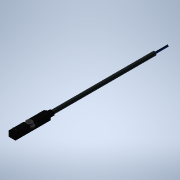
# Autodesk Inventor part: 574333 SMT-8M-A-1---OE---(part)
Saved by Autodesk Inventor 2021 (Build 250183000, 183)
## iProperties
Created: 2026-04-08
Part Number: 574333 SMT-8M-A-1---OE---(part)
Material: Generic
Catalog Web Link: www.3dfindit.com
Description: SMT-8M-A_part-Proximity switch
Vendor: FESTO
Document SubType Name: Modeling
Designer: psAdmin
Manufacturer: FESTO
Mass: 1.11911 g
Surface Area: 14.2957 cm^2
Volume: 1.11911 cm^3
Density: 1 g/cm^3
Appearance: PSOLRGB-176-176-176
Category: PARTsolutions
Company: FESTO
Title: 574333 SMT-8M-A-1---OE---(part)
Author: Cadenas PARTsolutions
Comments: Proximity switch
PSOL_IDENT_0: {$CADENAS_DATA/23d-libs/festo/parts/s/smt/parts/smt_8m_a.prj},219 {VTYP=3D},{NB=574333 SMT-8M-A-1---
PSOL_IDENT_1: OE---(part)},{LINA=574333 SMT-8M-A-1---OE---(part)},{NN=SMT-8M-A_part},{DATE=22.11.2021 21:11:07},{G
PSOL_IDENT_2: EOMDATE=22.11.2021 21:11:00},{VERSION=},{LINEID=10},{WBVAR=SA,LB,AT},{WBNUMERIC=SA}  {NB=574333 SMT-
PSOL_IDENT_3: 8M-A-1---OE---(part)},{LINA=574333 SMT-8M-A-1---OE---(part)},{KT=DUMMY},{TNR=574333},{TYP=SMT-8M-A},
PSOL_IDENT_4: {SA=1},{LB=-},{AT=OE}
NB: 574333 SMT-8M-A-1---OE---(part)
NN: SMT-8M-A_part
NT: Proximity switch
NBSYN: $TNR. $TYP.-$SA.-$LB.-$AT.---(part)
LINA: 574333 SMT-8M-A-1---OE---(part)
CATALOG: Festo
TNR: 574333
TYP: SMT-8M-A
SA: PS
LB: -
AT: OE
SUPPLIER: FESTO
ARTICLENO: 574333 SMT-8M-A-1---OE---(part)
BOMINFO: 574333 SMT-8M-A-1---OE---(part)
CREATOR: CADENAS GmbH
Autodesk Inventor part; units mm, degrees
sketch "Sketch_1" plane through (0, 0, 0) normal (0, 0, 1) x (1, 0, 0)
  line L0 (-2.5, 4.0386) -> (-2.5, 0)
  line L1 (-2.5, 0) -> (2.5, 0)
  line L2 (2.5, 0) -> (2.5, 4.0386)
  arc A0 (2.5, 4.0386) -> (2.3613, 4.229) centre (2.3, 4.0386) ccw
  arc A1 (2.3613, 4.229) -> (-2.3613, 4.229) centre (0, -3.1) ccw
  arc A2 (-2.3613, 4.229) -> (-2.5, 4.0386) centre (-2.3, 4.0386) ccw
  constraints: 6 end point, 6 point on circle, 3 centre point
extrude "Extrusion1" add sketch "Sketch_1" along normal blind 26.3
sketch "Sketch_2" plane through (-1.6, 0, 0) normal (1, 0, 0) x (0, 0, -1)
  line L0 (-15.3, 3.85) -> (-15.3, 2)
  line L1 (-15.3, 2) -> (-10.025, 2)
  line L2 (-10.025, 2) -> (-10.025, 3.15)
  line L3 (-10.025, 3.15) -> (-10.725, 3.15)
  line L4 (-10.725, 3.15) -> (-10.725, 3.85)
  line L5 (-10.725, 3.85) -> (-15.3, 3.85)
  constraints: 12 end point
extrude "Extrusion2" cut sketch "Sketch_2" along normal blind 4.1
sketch "Sketch_3" plane through (-2.5, 0, 0) normal (1, 0, 0) x (0, 0, -1)
  line L0 (-16.875, 3.85) -> (-16.875, 2)
  line L1 (-16.875, 2) -> (-11.6, 2)
  line L2 (-11.6, 2) -> (-11.6, 3.85)
  line L3 (-11.6, 3.85) -> (-16.875, 3.85)
  constraints: 8 end point
extrude "Extrusion3" cut sketch "Sketch_3" along normal blind 4.1
sketch "Sketch_4" plane through (0, 4.6, 0) normal (0, 1, 0) x (1, 0, 0)
  line L0 (-3, -15.3) -> (-1.3666, -15.3)
  arc A0 (-1.3666, -15.3) -> (1.3666, -15.3) centre (0, -13.45) ccw
  line L1 (1.3666, -15.3) -> (3, -15.3)
  line L2 (3, -15.3) -> (3, -11.6)
  line L3 (3, -11.6) -> (1.3666, -11.6)
  arc A1 (1.3666, -11.6) -> (-1.3666, -11.6) centre (0, -13.45) ccw
  line L4 (-1.3666, -11.6) -> (-3, -11.6)
  line L5 (-3, -11.6) -> (-3, -15.3)
  constraints: 12 end point, 4 point on circle, 2 centre point
extrude "Extrusion4" cut sketch "Sketch_4" against normal blind 2.5
sketch "Sketch_5" plane through (0, 2, 0) normal (0, 1, 0) x (1, 0, 0)
  arc A0 (-2.6719, -11.644) -> (-2.6719, -15.256) centre (0, -13.45) ccw
  arc A1 (-2.6719, -15.256) -> (-2.589, -15.3) centre (-2.589, -15.2) ccw
  line L0 (-2.589, -15.3) -> (-1.9442, -15.3)
  arc A2 (-1.6255, -15.4148) -> (-1.9442, -15.3) centre (-1.9442, -15.8) ccw
  arc A3 (-1.6255, -15.4148) -> (1.6255, -15.4148) centre (0, -13.45) ccw
  arc A4 (1.9442, -15.3) -> (1.6255, -15.4148) centre (1.9442, -15.8) ccw
  line L1 (1.9442, -15.3) -> (2.589, -15.3)
  arc A5 (2.589, -15.3) -> (2.6719, -15.256) centre (2.589, -15.2) ccw
  arc A6 (2.6719, -15.256) -> (2.6719, -11.644) centre (0, -13.45) ccw
  arc A7 (2.6719, -11.644) -> (2.589, -11.6) centre (2.589, -11.7) ccw
  line L2 (2.589, -11.6) -> (1.9442, -11.6)
  arc A8 (1.6255, -11.4852) -> (1.9442, -11.6) centre (1.9442, -11.1) ccw
  arc A9 (1.6255, -11.4852) -> (-1.6255, -11.4852) centre (0, -13.45) ccw
  arc A10 (-1.9442, -11.6) -> (-1.6255, -11.4852) centre (-1.9442, -11.1) ccw
  line L3 (-1.9442, -11.6) -> (-2.589, -11.6)
  arc A11 (-2.589, -11.6) -> (-2.6719, -11.644) centre (-2.589, -11.7) ccw
  constraints: 24 point on circle, 12 centre point, 8 end point
extrude "Extrusion5" add sketch "Sketch_5" along normal blind 1
sketch "Sketch_6" plane through (0, 0, 13.45) normal (0, 0, 1) x (1, 0, 0)
  line L0 (0, 2) -> (0, 4.6)
  line L1 (0, 4.6) -> (2.25, 4.6)
  line L2 (2.25, 4.6) -> (2.25, 3.9)
  line L3 (2.25, 3.9) -> (1.6935, 3.9)
  line L4 (1.6935, 3.9) -> (1.6935, 3.6)
  line L5 (1.6935, 3.6) -> (2, 3.2935)
  line L6 (2, 3.2935) -> (2, 2.3065)
  line L7 (2, 2.3065) -> (1.6935, 2)
  line L8 (1.6935, 2) -> (0, 2)
  line L9 (0, 2) -> (0, 4.6)
  constraints: 20 end point
revolve "Revolution1" add sketch "Sketch_6" angle 360 about axis through (0, 2, 13.45) along (0, -1, 0)
thread "Thread1" size "M4x0.5" class "6g" standard "ISO Metric profile" length 0.987
sketch "Sketch_7" plane through (0, 4.6, 13.45) normal (0, 1, 0) x (1, 0, 0)
  line L0 (-0.75, -0.433) -> (0, -0.866)
  line L1 (0, -0.866) -> (0.75, -0.433)
  line L2 (0.75, -0.433) -> (0.75, 0.433)
  line L3 (0.75, 0.433) -> (0, 0.866)
  line L4 (0, 0.866) -> (-0.75, 0.433)
  line L5 (-0.75, 0.433) -> (-0.75, -0.433)
  constraints: 12 end point
extrude "Extrusion6" cut sketch "Sketch_7" against normal blind 1.4
sketch "Sketch_9" plane through (0, 0, 23.21) normal (0, 0, 1) x (1, 0, 0)
  line L0 (-2.5, 2.8) -> (2.5, 2.8)
  line L1 (2.5, 2.8) -> (2.5, 4.2485)
  arc A0 (2.5, 4.2485) -> (2.3597, 4.4393) centre (2.3, 4.2485) ccw
  arc A1 (2.3597, 4.4393) -> (-2.3597, 4.4393) centre (0, -3.1) ccw
  arc A2 (-2.3597, 4.4393) -> (-2.5, 4.2485) centre (-2.3, 4.2485) ccw
  line L2 (-2.5, 4.2485) -> (-2.5, 2.8)
  constraints: 6 end point, 6 point on circle, 3 centre point
extrude "Extrusion7" add sketch "Sketch_9" along normal mid plane 0.4
sketch "Sketch_10" plane through (0, 0, 23.21) normal (0, 0, 1) x (1, 0, 0)
  line L0 (-0.2, 2.78) -> (0.2, 2.78)
  line L1 (0.2, 2.78) -> (0.2, 4.78)
  line L2 (0.2, 4.78) -> (-0.2, 4.78)
  line L3 (-0.2, 4.78) -> (-0.2, 2.78)
  constraints: 8 end point
extrude "Extrusion8" add sketch "Sketch_10" along normal mid plane 2
sketch "Sketch_11" plane through (0, 0, 0) normal (1, 0, 0) x (0, 1, 0)
  line L0 (2.05, -90) -> (2.05, 0)
  line L1 (2.05, 0) -> (4.05, 0)
  line L2 (4.05, 0) -> (4.05, -3)
  line L3 (4.05, -3) -> (3.5, -3)
  line L4 (3.5, -3) -> (3.5, -90)
  line L5 (3.5, -90) -> (2.05, -90)
  line L6 (2.05, -90) -> (2.05, 0)
  constraints: 14 end point
revolve "Revolution2" add sketch "Sketch_11" angle 360 about axis through (0, 2.05, -90) along (0, 0, -1)
sketch "Sketch_12" plane through (0, 2.05, -90) normal (0, 0, -1) x (0, 1, 0)
  line L0 (-2, -2) -> (2, -2)
  line L1 (2, -2) -> (2, 2)
  line L2 (2, 2) -> (-2, 2)
  line L3 (-2, 2) -> (-2, -2)
  circle A0 centre (0.4, 0) radius 0.3
  circle A1 centre (-0.2, 0.3464) radius 0.3
  circle A2 centre (-0.2, -0.3464) radius 0.3
  constraints: 8 end point, 3 centre point
extrude "Extrusion9" cut sketch "Sketch_12" against normal blind 10
sketch "Sketch_17" plane through (0, 0, -1.5) normal (0, 0, 1) x (1, 0, 0)
  arc A0 (-3.0691, 2.4416) -> (-2.9069, 2.2099) centre (-2.8722, 2.4069) ccw
  line L0 (-2.9069, 2.2099) -> (0, 1.6973)
  line L1 (0, 1.6973) -> (2.9069, 2.2099)
  arc A1 (2.9069, 2.2099) -> (3.0691, 2.4416) centre (2.8722, 2.4069) ccw
  line L2 (3.0691, 2.4416) -> (3.0531, 2.5326)
  arc A2 (3.0531, 2.5326) -> (2.8214, 2.6948) centre (2.8561, 2.4979) ccw
  line L3 (2.8214, 2.6948) -> (0, 2.1973)
  line L4 (0, 2.1973) -> (-2.8214, 2.6948)
  arc A3 (-2.8214, 2.6948) -> (-3.0531, 2.5326) centre (-2.8561, 2.4979) ccw
  line L5 (-3.0531, 2.5326) -> (-3.0691, 2.4416)
  constraints: 12 end point, 8 point on circle, 4 centre point
extrude "Extrusion10" add sketch "Sketch_17" along normal mid plane 1.8
ref_plane "ANBAU_XY" through (0, 0, 0) normal (0, 0, -1) x (1, 0, 0)
ref_plane "ANBAU_YZ" through (0, 0, 0) normal (1, 0, 0) x (0, -1, 0)
ref_plane "ANBAU_ZX" through (0, 0, 0) normal (0, -1, 0) x (0, 0, -1)
ref_plane "ASCF1_XY" through (0, 2.05, -10) normal (0, 0, -1) x (1, 0, 0)
ref_plane "ASCF1_YZ" through (0, 2.05, -10) normal (1, 0, 0) x (0, -1, 0)
ref_plane "ASCF1_ZX" through (0, 2.05, -10) normal (0, -1, 0) x (0, 0, -1)
ref_plane "ASCF2_XY" through (0, 2.05, -75) normal (0, 0, 1) x (1, 0, 0)
ref_plane "ASCF2_YZ" through (0, 2.05, -75) normal (1, 0, 0) x (0, 1, 0)
ref_plane "ASCF2_ZX" through (0, 2.05, -75) normal (0, 1, 0) x (0, 0, 1)
ref_plane "FDT_NUT_XY" through (0, 0, 26.3) normal (0, -1, 0) x (1, 0, 0)
ref_plane "FDT_NUT_YZ" through (0, 0, 26.3) normal (1, 0, 0) x (0, 0, 1)
ref_plane "FDT_NUT_ZX" through (0, 0, 26.3) normal (0, 0, 1) x (0, -1, 0)
body "Solid1"
